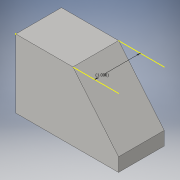
# Autodesk Inventor part: A2.6_Titus_SketchSheetA9
Saved by Autodesk Inventor 2016 (Build 200138000, 138)
## iProperties
Created: 2017-09-15
Part Number: A2.6_Titus_SketchSheetA9
Material: Generic
Document SubType Name: Modeling
Designer: sun01147
Density: 1 g/cm^3
Appearance: Default
Author: sun01147
Autodesk Inventor part; units mm, degrees
ref_plane "YZ Plane" through (0, 0, 0) normal (1, 0, 0) x (0, 1, 0)
ref_plane "XZ Plane" through (0, 0, 0) normal (0, 1, 0) x (-1, 0, 0)
ref_plane "XY Plane" through (0, 0, 0) normal (0, 0, 1) x (1, 0, 0)
sketch "Sketch1" plane through (0, 0, 0) normal (0, 0, 1) x (1, 0, 0)
  line L0 (0, 0) -> (57.15, 0)
  line L1 (57.15, 0) -> (57.15, 38.1)
  line L2 (57.15, 38.1) -> (0, 38.1)
  line L3 (0, 38.1) -> (0, 0)
  line L4 (31.75, 38.1) -> (57.15, 7.525)
  dimension "d0" = 38.1
  dimension "d1" = 57.15
  dimension "d2" = 30.575
  dimension "d3" = 25.4
  constraints: 10 end point, 2 parallel, 2 point on line, 1 horizontal, 1 perpendicular
  measures "d0" distance of L2.end L0.start
  measures "d1" distance of L1.end L2.end
  measures "d2" vertical distance of L4.start L4.end
  measures "d3" horizontal distance of L4.start L4.end
extrude "Extrusion1" add sketch "Sketch1" against normal blind 25.4 contours L3 L2 L4 L1 L0
sketch "Sketch2" plane through (0, 38.1, 0) normal (0, 1, 0) x (1, 0, 0)
  line L0 (31.75, 25.4) -> (57.15, 25.4) projected
  line L1 (57.15, 0) -> (31.75, 0) projected
  point P0 (0, 0)
  dimension "d6" = 25.4
  measures "d6" distance between parallel lines of L0 L1
body "Solid1"
